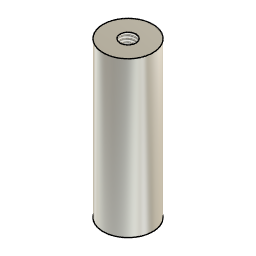
Aluminum Bar φ8 x 25mm (Autodesk Fusion 360 design; units mm, degrees)
Autodesk Fusion 360 part; units mm, degrees
sketch "スケッチ1" plane through (0, 0, 0) normal (0, 0, 1) x (1, 0, 0)
  circle A0 centre (0, 0) radius 4
  dimension "d1" = 8
  constraint coincident A0.centre origin
  measures "d1" diameter of A0
extrude "押し出し1" add sketch "スケッチ1" along normal blind 25
cylinder "円柱プリミティブ2" cut diameter 3 height -5 placed x (1, 0, 0) y (0, 1, 0) z (0, 0, 1) at (0, 0, 25)
thread "ねじ2" "ISO Metric profile 3.0 M3x0.5 6H" major diameter 3.086 minor diameter 2.529 pitch 0.5 angle 60 resizes the face on face at (1.4925, -0.1494, 23.3333)
cylinder "円柱プリミティブ3" cut diameter 3 height -5 placed x (0, 1, 0) y (1, 0, 0) z (0, 0, -1) at (0, 0, 0)
thread "ねじ3" "ISO Metric profile 3.0 M3x0.5 6H" major diameter 3.086 minor diameter 2.529 pitch 0.5 angle 60 resizes the face on face at (-0.1494, 1.4925, 1.6667)
